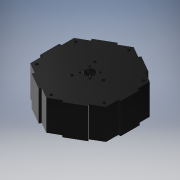
# Autodesk Inventor part: Spur Gear2
Saved by Autodesk Inventor 2017 (Build 210142000, 142)
## iProperties
Created: 2018-10-09
Part Number: Spur Gear2
Material: ABS Plastic
Document SubType Name: Modeling
Designer: Zach
Categories: <?xml version="1.0" encoding="UTF-16"?> <MemberInstance><Categories><FamilyTemplate><FamilyTemplateParameter ValueType="xs:double" Id="1" ObjectReferenceKey="da_z" ObjectType="kUserParameterObject"/><FamilyTemplateParameter ValueType="xs:double" Id="2" ObjectReferenceKey="da_b" ObjectType="kUserParameterObject"/><FamilyTemplateParameter ValueType="xs:double" Id="3" ObjectReferenceKey="da_beta" ObjectType="kUserParameterObject"/><FamilyTemplateParameter ValueType="xs:double" Id="4" ObjectReferenceKey="da_da" ObjectType="kUserParameterObject"/><FamilyTemplateParameter ValueType="xs:double" Id="5" ObjectReferenceKey="da_aw" ObjectType="kUserParameterObject"/><FamilyTemplateParameter ValueType="xs:string" Id="6" ObjectReferenceKey="EAIAABAAAACIAQAAAAAAAIAAAAAAAAAA" ObjectType="83910656" SubObjectId="SurfaceGeometry"/></FamilyTemplate><ParamToTemplateMap><ParamToTemplate CategoryParameter="//CategoryParameter[@InternalName='046C89C9-8512-4d59-83FE-43B91F4F132A']" TemplateParameter="1"/><ParamToTemplate CategoryParameter="//CategoryParameter[@InternalName='2552DF32-E462-4b46-AEBF-C6C7768E72AC']" TemplateParameter="2"/><ParamToTemplate CategoryParameter="//CategoryParameter[@InternalName='C9EE641D-15FC-4fae-A226-E94C4372FDD7']" TemplateParameter="3"/><ParamToTemplate><ParamToTemplate CategoryParameter="//CategoryParameter[@InternalName='00B6519A-459B-49c7-AD84-2E56D39A5744']" ConstantValue="0.000000"/></ParamToTemplate><ParamToTemplate><ParamToTemplate CategoryParameter="//CategoryParameter[@InternalName='04B31F0E-C7A6-4894-AA32-9629BEFACF47']" ConstantValue="1.000000"/></ParamToTemplate><ParamToTemplate><ParamToTemplate CategoryParameter="//CategoryParameter[@InternalName='43CBEC2E-7847-49e7-A936-2F7889FCB2D9']" ConstantValue="0.250000"/></ParamToTemplate><ParamToTemplate><ParamToTemplate CategoryParameter="//CategoryParameter[@InternalName='B1EFC894-105D-4ebd-86BF-FA20ED196853']" ConstantValue="0.350000"/></ParamToTemplate><ParamToTemplate><ParamToTemplate CategoryParameter="//CategoryParameter[@InternalName='51175063-3D10-4879-93E8-6246FE8B403D']" ConstantValue="2060000000.000000"/></ParamToTemplate><ParamToTemplate><ParamToTemplate CategoryParameter="//CategoryParameter[@InternalName='A3A52E27-4454-46a9-B0BD-C932399B70AF']" ConstantValue="0.300000"/></ParamToTemplate><ParamToTemplate><ParamToTemplate CategoryParameter="//CategoryParameter[@InternalName='91B76062-C214-41d9-B1B9-14D2AB99603D']" ConstantValue="0.200000"/></ParamToTemplate><ParamToTemplate><ParamToTemplate CategoryParameter="//CategoryParameter[@InternalName='374E806E-8B8A-4dda-A9AA-1039D6500AD2']" ConstantValue="5.000000"/></ParamToTemplate><ParamToTemplate><ParamToTemplate CategoryParameter="//CategoryParameter[@InternalName='2D373A89-B862-43d6-8D0B-0CBF12AB9F6C']" ConstantValue="0.392699"/></ParamToTemplate><ParamToTemplate CategoryParameter="//CategoryParameter[@InternalName='37777632-D6A2-4fac-9D53-DB8ACD95C989']" TemplateParameter="4"/><ParamToTemplate CategoryParameter="//CategoryParameter[@InternalName='FD1017F1-B727-4f7e-9707-0F86F1FF9423']" TemplateParameter="5"/><ParamToTemplate><ParamToTemplate CategoryParameter="//CategoryParameter[@InternalName='9E1B4470-B2D3-4ff1-B813-535BB4CDF51A']" ConstantValue="3520000.000000"/></ParamToTemplate><ParamToTemplate><ParamToTemplate CategoryParameter="//CategoryParameter[@InternalName='F8452263-BFF6-458c-9FB1-07C4B99E95CD']" ConstantValue="11400000.000000"/></ParamToTemplate><ParamToTemplate><ParamToTemplate CategoryParameter="//CategoryParameter[@InternalName='3E3BB259-FD49-497f-8171-6EBC954A3479']" ConstantValue="2.000000"/></ParamToTemplate><ParamToTemplate CategoryParameter="//CategoryParameter[@InternalName='27C3BAF2-7550-4e4b-AE2C-0DB134B7D9B7']" TemplateParameter="6"/></ParamToTemplateMap><Category DisplayName="Gear" InternalName="DC85795E-93AB-48d5-8EEE-5A27447B64BD" Mnemonic="Gear"><CategoryParameter DisplayName="z" InternalName="046C89C9-8512-4d59-83FE-43B91F4F132A" Mnemonic="z"/><CategoryParameter DisplayName="b" InternalName="2552DF32-E462-4b46-AEBF-C6C7768E72AC" Mnemonic="b"/><CategoryParameter DisplayName="||b|" InternalName="C9EE641D-15FC-4fae-A226-E94C4372FDD7" Mnemonic="beta"/><CategoryParameter DisplayName="x" InternalName="00B6519A-459B-49c7-AD84-2E56D39A5744" Mnemonic="x"/><CategoryParameter DisplayName="a*" InternalName="04B31F0E-C7A6-4894-AA32-9629BEFACF47" Mnemonic="a"/><CategoryParameter DisplayName="c*" InternalName="43CBEC2E-7847-49e7-A936-2F7889FCB2D9" Mnemonic="c"/><CategoryParameter DisplayName="r|.f|*" InternalName="B1EFC894-105D-4ebd-86BF-FA20ED196853" Mnemonic="rf"/><CategoryParameter DisplayName="E" InternalName="51175063-3D10-4879-93E8-6246FE8B403D" Mnemonic="E"/><CategoryParameter DisplayName="||m|" InternalName="A3A52E27-4454-46a9-B0BD-C932399B70AF" Mnemonic="mi"/><Category DisplayName="SpurGear" InternalName="26C5A22E-A91E-4dfd-A3B3-23CCAFAE1764" Mnemonic="SpurGear"><CategoryParameter DisplayName="m" InternalName="91B76062-C214-41d9-B1B9-14D2AB99603D" Mnemonic="m"/><CategoryParameter DisplayName="P" InternalName="374E806E-8B8A-4dda-A9AA-1039D6500AD2" Mnemonic="PP"/><CategoryParameter DisplayName="||a|" InternalName="2D373A89-B862-43d6-8D0B-0CBF12AB9F6C" Mnemonic="alpha"/><CategoryParameter DisplayName="d|.a|" InternalName="37777632-D6A2-4fac-9D53-DB8ACD95C989" Mnemonic="da"/><CategoryParameter DisplayName="a|.w|" InternalName="FD1017F1-B727-4f7e-9707-0F86F1FF9423" Mnemonic="aw"/><CategoryParameter DisplayName="||s||.Flim|" InternalName="9E1B4470-B2D3-4ff1-B813-535BB4CDF51A" Mnemonic="sFlim"/><CategoryParameter DisplayName="||s||.Hlim|" InternalName="F8452263-BFF6-458c-9FB1-07C4B99E95CD" Mnemonic="sHlim"/><CategoryParameter DisplayName="type" InternalName="3E3BB259-FD49-497f-8171-6EBC954A3479" Mnemonic="type"/><Category DisplayName="InternalSpurGear" InternalName="7CF704F6-14A9-42f8-93CE-E71DF57C2B55" Mnemonic="InternalSpurGear"><CategoryParameter DisplayName="PitchDiameter" InternalName="27C3BAF2-7550-4e4b-AE2C-0DB134B7D9B7" Mnemonic="IDS_PITCHDIAM"/></Category></Category></Category></Categories></MemberInstance>
Density: 1.06 g/cm^3
Appearance: Smooth - Black
Mass: 196.31 g
Surface Area: 506.785 cm^2
Volume: 185.198 cm^3
CustomPartVersion: 0
Author: Zach
Autodesk Inventor part; units mm, degrees
ref_plane "YZ Plane" through (0, 0, 0) normal (1, 0, 0) x (0, 1, 0)
ref_plane "XZ Plane" through (0, 0, 0) normal (0, 1, 0) x (-1, 0, 0)
ref_plane "XY Plane" through (0, 0, 0) normal (0, 0, 1) x (1, 0, 0)
sketch "Sketch1" plane through (0, 0, 0) normal (0, 0, 1) x (1, 0, 0)
  circle A0 centre (0, 0) radius 52.25
  dimension "d0" = 104.5
  constraints: 1 centre point
  measures "d0" diameter of A0
extrude "Extrusion1" add sketch "Sketch1" along normal blind 10
ref_plane "Work Plane2" through (0, 0, 5) normal (0, 0, 1) x (1, 0, 0)
sketch "Sketch2" plane through (0, 0, 0) normal (0, 0, -1) x (-1, 0, 0)
  circle A0 centre (0, 0) radius 52.25 projected
  circle A1 centre (0, 0) radius 45
  dimension "d3" = 90
  constraints: 1 centre point, 1 coincident
  measures "d3" diameter of A1
surface extrude "Pitch Diameter" sketch "Sketch2" against normal through all shown no curves A1
ref_plane "Work Plane8" through (0, 0, 0) normal (0.9975641, 0.0697565, 0) x (0, 0, 1)
ref_plane "Work Plane9" through (0, 0, 0) normal (1, 0, 0) x (0, 1, 0)
spur gear teeth "Spur Gear" teeth 45 pitch diameter 90 tip diameter 86.2612 root diameter 95 face width 10 start plane through (0, 0, 0) normal (0, 0, -1) x (-1, 0, 0)
sketch "Sketch3" plane through (0, 0, 10) normal (0, 0, 1) x (1, 0, 0)
  arc A0 (2.2573, -43.0715) -> (3.7591, -42.9665) centre (0, 0) ccw projected
  arc A1 (0.829, -47.4928) -> (2.2573, -43.0715) centre (-19.4558, -38.4984) ccw projected
  arc A2 (-0.829, -47.4928) -> (0.829, -47.4928) centre (0, 0) ccw projected
  arc A3 (-2.2573, -43.0715) -> (-0.829, -47.4928) centre (19.4558, -38.4984) ccw projected
  arc A4 (-3.7591, -42.9665) -> (-2.2573, -43.0715) centre (0, 0) ccw projected
  arc A5 (-5.7888, -47.1459) -> (-3.7591, -42.9665) centre (-24.6244, -35.4161) ccw projected
  arc A6 (-7.4306, -46.9152) -> (-5.7888, -47.1459) centre (0, 0) ccw projected
  arc A7 (-8.2297, -42.3382) -> (-7.4306, -46.9152) centre (13.9085, -40.8315) ccw projected
  arc A8 (-9.7023, -42.0252) -> (-8.2297, -42.3382) centre (0, 0) ccw projected
  arc A9 (-12.2939, -45.8815) -> (-9.7023, -42.0252) centre (-29.3137, -31.6443) ccw projected
  arc A10 (-13.8877, -45.4245) -> (-12.2939, -45.8815) centre (0, 0) ccw projected
  arc A11 (-14.0419, -40.7808) -> (-13.8877, -45.4245) centre (8.0905, -42.3698) ccw projected
  arc A12 (-15.4566, -40.2659) -> (-14.0419, -40.7808) centre (0, 0) ccw projected
  arc A13 (-18.5597, -43.724) -> (-15.4566, -40.2659) centre (-33.4325, -27.2567) ccw projected
  arc A14 (-20.0744, -43.0496) -> (-18.5597, -43.724) centre (0, 0) ccw projected
  arc A15 (-19.5809, -38.4296) -> (-20.0744, -43.0496) centre (2.115, -43.0835) ccw projected
  arc A16 (-20.9101, -37.7229) -> (-19.5809, -38.4296) centre (0, 0) ccw projected
  arc A17 (-24.4643, -40.7154) -> (-20.9101, -37.7229) centre (-36.9005, -22.3385) ccw projected
  arc A18 (-25.8704, -39.8369) -> (-24.4643, -40.7154) centre (0, 0) ccw projected
  arc A19 (-24.7387, -35.3305) -> (-25.8704, -39.8369) centre (-3.9016, -42.9585) ccw projected
  arc A20 (-25.9566, -34.4456) -> (-24.7387, -35.3305) centre (0, 0) ccw projected
  arc A21 (-29.8927, -36.9144) -> (-25.9566, -34.4456) centre (-39.6503, -16.9856) ccw projected
  arc A22 (-31.1628, -35.8487) -> (-29.8927, -36.9144) centre (0, 0) ccw projected
  arc A23 (-29.415, -31.5437) -> (-31.1628, -35.8487) centre (-9.8423, -41.9975) ccw projected
  arc A24 (-30.4979, -30.4979) -> (-29.415, -31.5437) centre (0, 0) ccw projected
  arc A25 (-34.7393, -32.3949) -> (-30.4979, -30.4979) centre (-41.6284, -11.302) ccw projected
  arc A26 (-35.8487, -31.1628) -> (-34.7393, -32.3949) centre (0, 0) ccw projected
  arc A27 (-33.5188, -27.143) -> (-35.8487, -31.1628) centre (-15.5915, -40.219) ccw projected
  arc A28 (-34.4456, -25.9566) -> (-33.5188, -27.143) centre (0, 0) ccw projected
  arc A29 (-38.9097, -27.2449) -> (-34.4456, -25.9566) centre (-42.7962, -5.3985) ccw projected
  arc A30 (-39.8369, -25.8704) -> (-38.9097, -27.2449) centre (0, 0) ccw projected
  arc A31 (-36.9701, -22.2139) -> (-39.8369, -25.8704) centre (-21.0371, -37.6576) ccw projected
  arc A32 (-37.7229, -20.9101) -> (-36.9701, -22.2139) centre (0, 0) ccw projected
  arc A33 (-42.3228, -21.5645) -> (-37.7229, -20.9101) centre (-43.131, 0.6101) ccw projected
  arc A34 (-43.0496, -20.0744) -> (-42.3228, -21.5645) centre (0, 0) ccw projected
  arc A35 (-39.7019, -16.8525) -> (-43.0496, -20.0744) centre (-26.0733, -34.3634) ccw projected
  arc A36 (-40.2659, -15.4566) -> (-39.7019, -16.8525) centre (0, 0) ccw projected
  arc A37 (-44.9121, -15.4645) -> (-40.2659, -15.4566) centre (-42.6264, 6.6069) ccw projected
  arc A38 (-45.4245, -13.8877) -> (-44.9121, -15.4645) centre (0, 0) ccw projected
  arc A39 (-41.6609, -11.163) -> (-45.4245, -13.8877) centre (-30.602, -30.4002) ccw projected
  arc A40 (-42.0252, -9.7023) -> (-41.6609, -11.163) centre (0, 0) ccw projected
  arc A41 (-46.6273, -9.0634) -> (-42.0252, -9.7023) centre (-41.292, 12.475) ccw projected
  arc A42 (-46.9152, -7.4306) -> (-46.6273, -9.0634) centre (0, 0) ccw projected
  arc A43 (-42.8091, -5.2563) -> (-46.9152, -7.4306) centre (-34.5351, -25.8454) ccw projected
  arc A44 (-42.9665, -3.7591) -> (-42.8091, -5.2563) centre (0, 0) ccw projected
  arc A45 (-47.4349, -2.486) -> (-42.9665, -3.7591) centre (-39.154, 18.1004) ccw projected
  arc A46 (-47.4928, -0.829) -> (-47.4349, -2.486) centre (0, 0) ccw projected
  arc A47 (-43.124, 0.7527) -> (-47.4928, -0.829) centre (-37.796, -20.7875) ccw projected
  arc A48 (-43.0715, 2.2573) -> (-43.124, 0.7527) centre (0, 0) ccw projected
  arc A49 (-47.3192, 4.1399) -> (-43.0715, 2.2573) centre (-36.2539, 23.3734) ccw projected
  arc A50 (-47.1459, 5.7888) -> (-47.3192, 4.1399) centre (0, 0) ccw projected
  arc A51 (-42.5996, 6.7471) -> (-47.1459, 5.7888) centre (-40.3212, -15.325) ccw projected
  arc A52 (-42.3382, 8.2297) -> (-42.5996, 6.7471) centre (0, 0) ccw projected
  arc A53 (-46.2826, 10.6852) -> (-42.3382, 8.2297) centre (-32.6481, 28.1915) ccw projected
  arc A54 (-45.8815, 12.2939) -> (-46.2826, 10.6852) centre (0, 0) ccw projected
  arc A55 (-41.246, 12.6102) -> (-45.8815, 12.2939) centre (-42.0617, -9.5642) ccw projected
  arc A56 (-40.7808, 14.0419) -> (-41.246, 12.6102) centre (0, 0) ccw projected
  arc A57 (-44.3451, 17.0225) -> (-40.7808, 14.0419) centre (-28.4069, 32.4609) ccw projected
  arc A58 (-43.724, 18.5597) -> (-44.3451, 17.0225) centre (0, 0) ccw projected
  arc A59 (-39.0896, 18.2278) -> (-43.724, 18.5597) centre (-42.9834, -3.6173) ccw projected
  arc A60 (-38.4296, 19.5809) -> (-39.0896, 18.2278) centre (0, 0) ccw projected
  arc A61 (-41.5444, 23.0285) -> (-38.4296, 19.5809) centre (-23.6127, 36.0984) ccw projected
  arc A62 (-40.7154, 24.4643) -> (-41.5444, 23.0285) centre (0, 0) ccw projected
  arc A63 (-36.1724, 23.4906) -> (-40.7154, 24.4643) centre (-43.0685, 2.4) ccw projected
  arc A64 (-35.3305, 24.7387) -> (-36.1724, 23.4906) centre (0, 0) ccw projected
  arc A65 (-37.9352, 28.5862) -> (-35.3305, 24.7387) centre (-18.359, 39.0334) ccw projected
  arc A66 (-36.9144, 29.8927) -> (-37.9352, 28.5862) centre (0, 0) ccw projected
  arc A67 (-32.5511, 28.2962) -> (-36.9144, 29.8927) centre (-42.3154, 8.3706) ccw projected
  arc A68 (-31.5437, 29.415) -> (-32.5511, 28.2962) centre (0, 0) ccw projected
  arc A69 (-33.5876, 33.5876) -> (-31.5437, 29.415) centre (-12.748, 41.2086) ccw projected
  arc A70 (-32.3949, 34.7393) -> (-33.5876, 33.5876) centre (0, 0) ccw projected
  arc A71 (-28.2962, 32.5511) -> (-32.3949, 34.7393) centre (-40.7386, 14.1783) ccw projected
  arc A72 (-27.143, 33.5188) -> (-28.2962, 32.5511) centre (0, 0) ccw projected
  arc A73 (-28.5862, 37.9352) -> (-27.143, 33.5188) centre (-6.8888, 42.5817) ccw projected
  arc A74 (-27.2449, 38.9097) -> (-28.5862, 37.9352) centre (0, 0) ccw projected
  arc A75 (-23.4906, 36.1724) -> (-27.2449, 38.9097) centre (-38.3689, 19.7101) ccw projected
  arc A76 (-22.2139, 36.9701) -> (-23.4906, 36.1724) centre (0, 0) ccw projected
  arc A77 (-23.0285, 41.5444) -> (-22.2139, 36.9701) centre (-0.8955, 43.126) ccw projected
  arc A78 (-21.5645, 42.3228) -> (-23.0285, 41.5444) centre (0, 0) ccw projected
  arc A79 (-18.2278, 39.0896) -> (-21.5645, 42.3228) centre (-35.2524, 24.8582) ccw projected
  arc A80 (-16.8525, 39.7019) -> (-18.2278, 39.0896) centre (0, 0) ccw projected
  arc A81 (-17.0225, 44.3451) -> (-16.8525, 39.7019) centre (5.1152, 42.831) ccw projected
  arc A82 (-15.4645, 44.9121) -> (-17.0225, 44.3451) centre (0, 0) ccw projected
  arc A83 (-12.6102, 41.246) -> (-15.4645, 44.9121) centre (-31.4497, 29.5224) ccw projected
  arc A84 (-11.163, 41.6609) -> (-12.6102, 41.246) centre (0, 0) ccw projected
  arc A85 (-10.6852, 46.2826) -> (-11.163, 41.6609) centre (11.0263, 41.7022) ccw projected
  arc A86 (-9.0634, 46.6273) -> (-10.6852, 46.2826) centre (0, 0) ccw projected
  arc A87 (-6.7471, 42.5996) -> (-9.0634, 46.6273) centre (-27.0349, 33.6121) ccw projected
  arc A88 (-5.2563, 42.8091) -> (-6.7471, 42.5996) centre (0, 0) ccw projected
  arc A89 (-4.1399, 47.3192) -> (-5.2563, 42.8091) centre (16.7229, 39.7618) ccw projected
  arc A90 (-2.486, 47.4349) -> (-4.1399, 47.3192) centre (0, 0) ccw projected
  arc A91 (-0.7527, 43.124) -> (-2.486, 47.4349) centre (-22.0939, 37.0475) ccw projected
  arc A92 (0.7527, 43.124) -> (-0.7527, 43.124) centre (0, 0) ccw projected
  arc A93 (2.486, 47.4349) -> (0.7527, 43.124) centre (22.0939, 37.0475) ccw projected
  arc A94 (4.1399, 47.3192) -> (2.486, 47.4349) centre (0, 0) ccw projected
  arc A95 (5.2563, 42.8091) -> (4.1399, 47.3192) centre (-16.7229, 39.7618) ccw projected
  arc A96 (6.7471, 42.5996) -> (5.2563, 42.8091) centre (0, 0) ccw projected
  arc A97 (9.0634, 46.6273) -> (6.7471, 42.5996) centre (27.0349, 33.6121) ccw projected
  arc A98 (10.6852, 46.2826) -> (9.0634, 46.6273) centre (0, 0) ccw projected
  arc A99 (11.163, 41.6609) -> (10.6852, 46.2826) centre (-11.0263, 41.7022) ccw projected
  arc A100 (12.6102, 41.246) -> (11.163, 41.6609) centre (0, 0) ccw projected
  arc A101 (15.4645, 44.9121) -> (12.6102, 41.246) centre (31.4497, 29.5224) ccw projected
  arc A102 (17.0225, 44.3451) -> (15.4645, 44.9121) centre (0, 0) ccw projected
  arc A103 (16.8525, 39.7019) -> (17.0225, 44.3451) centre (-5.1152, 42.831) ccw projected
  arc A104 (18.2278, 39.0896) -> (16.8525, 39.7019) centre (0, 0) ccw projected
  arc A105 (21.5645, 42.3228) -> (18.2278, 39.0896) centre (35.2524, 24.8582) ccw projected
  arc A106 (23.0285, 41.5444) -> (21.5645, 42.3228) centre (0, 0) ccw projected
  arc A107 (22.2139, 36.9701) -> (23.0285, 41.5444) centre (0.8955, 43.126) ccw projected
  arc A108 (23.4906, 36.1724) -> (22.2139, 36.9701) centre (0, 0) ccw projected
  arc A109 (27.2449, 38.9097) -> (23.4906, 36.1724) centre (38.3689, 19.7101) ccw projected
  arc A110 (28.5862, 37.9352) -> (27.2449, 38.9097) centre (0, 0) ccw projected
  arc A111 (27.143, 33.5188) -> (28.5862, 37.9352) centre (6.8888, 42.5817) ccw projected
  arc A112 (28.2962, 32.5511) -> (27.143, 33.5188) centre (0, 0) ccw projected
  arc A113 (32.3949, 34.7393) -> (28.2962, 32.5511) centre (40.7386, 14.1783) ccw projected
  arc A114 (33.5876, 33.5876) -> (32.3949, 34.7393) centre (0, 0) ccw projected
  arc A115 (31.5437, 29.415) -> (33.5876, 33.5876) centre (12.748, 41.2086) ccw projected
  arc A116 (32.5511, 28.2962) -> (31.5437, 29.415) centre (0, 0) ccw projected
  arc A117 (36.9144, 29.8927) -> (32.5511, 28.2962) centre (42.3154, 8.3706) ccw projected
  arc A118 (37.9352, 28.5862) -> (36.9144, 29.8927) centre (0, 0) ccw projected
  arc A119 (35.3305, 24.7387) -> (37.9352, 28.5862) centre (18.359, 39.0334) ccw projected
  arc A120 (36.1724, 23.4906) -> (35.3305, 24.7387) centre (0, 0) ccw projected
  arc A121 (40.7154, 24.4643) -> (36.1724, 23.4906) centre (43.0685, 2.4) ccw projected
  arc A122 (41.5444, 23.0285) -> (40.7154, 24.4643) centre (0, 0) ccw projected
  arc A123 (38.4296, 19.5809) -> (41.5444, 23.0285) centre (23.6127, 36.0984) ccw projected
  arc A124 (39.0896, 18.2278) -> (38.4296, 19.5809) centre (0, 0) ccw projected
  arc A125 (43.724, 18.5597) -> (39.0896, 18.2278) centre (42.9834, -3.6173) ccw projected
  arc A126 (44.3451, 17.0225) -> (43.724, 18.5597) centre (0, 0) ccw projected
  arc A127 (40.7808, 14.0419) -> (44.3451, 17.0225) centre (28.4069, 32.4609) ccw projected
  arc A128 (41.246, 12.6102) -> (40.7808, 14.0419) centre (0, 0) ccw projected
  arc A129 (45.8815, 12.2939) -> (41.246, 12.6102) centre (42.0617, -9.5642) ccw projected
  arc A130 (46.2826, 10.6852) -> (45.8815, 12.2939) centre (0, 0) ccw projected
  arc A131 (42.3382, 8.2297) -> (46.2826, 10.6852) centre (32.6481, 28.1915) ccw projected
  arc A132 (42.5996, 6.7471) -> (42.3382, 8.2297) centre (0, 0) ccw projected
  arc A133 (47.1459, 5.7888) -> (42.5996, 6.7471) centre (40.3212, -15.325) ccw projected
  arc A134 (47.3192, 4.1399) -> (47.1459, 5.7888) centre (0, 0) ccw projected
  arc A135 (43.0715, 2.2573) -> (47.3192, 4.1399) centre (36.2539, 23.3734) ccw projected
  arc A136 (43.124, 0.7527) -> (43.0715, 2.2573) centre (0, 0) ccw projected
  arc A137 (47.4928, -0.829) -> (43.124, 0.7527) centre (37.796, -20.7875) ccw projected
  arc A138 (47.4349, -2.486) -> (47.4928, -0.829) centre (0, 0) ccw projected
  arc A139 (42.9665, -3.7591) -> (47.4349, -2.486) centre (39.154, 18.1004) ccw projected
  arc A140 (42.8091, -5.2563) -> (42.9665, -3.7591) centre (0, 0) ccw projected
  arc A141 (46.9152, -7.4306) -> (42.8091, -5.2563) centre (34.5351, -25.8454) ccw projected
  arc A142 (46.6273, -9.0634) -> (46.9152, -7.4306) centre (0, 0) ccw projected
  arc A143 (42.0252, -9.7023) -> (46.6273, -9.0634) centre (41.292, 12.475) ccw projected
  arc A144 (41.6609, -11.163) -> (42.0252, -9.7023) centre (0, 0) ccw projected
  arc A145 (45.4245, -13.8877) -> (41.6609, -11.163) centre (30.602, -30.4002) ccw projected
  arc A146 (44.9121, -15.4645) -> (45.4245, -13.8877) centre (0, 0) ccw projected
  arc A147 (40.2659, -15.4566) -> (44.9121, -15.4645) centre (42.6264, 6.6069) ccw projected
  arc A148 (39.7019, -16.8525) -> (40.2659, -15.4566) centre (0, 0) ccw projected
  arc A149 (43.0496, -20.0744) -> (39.7019, -16.8525) centre (26.0733, -34.3634) ccw projected
  arc A150 (42.3228, -21.5645) -> (43.0496, -20.0744) centre (0, 0) ccw projected
  arc A151 (37.7229, -20.9101) -> (42.3228, -21.5645) centre (43.131, 0.6101) ccw projected
  arc A152 (36.9701, -22.2139) -> (37.7229, -20.9101) centre (0, 0) ccw projected
  arc A153 (39.8369, -25.8704) -> (36.9701, -22.2139) centre (21.0371, -37.6576) ccw projected
  arc A154 (38.9097, -27.2449) -> (39.8369, -25.8704) centre (0, 0) ccw projected
  arc A155 (34.4456, -25.9566) -> (38.9097, -27.2449) centre (42.7962, -5.3985) ccw projected
  arc A156 (33.5188, -27.143) -> (34.4456, -25.9566) centre (0, 0) ccw projected
  arc A157 (35.8487, -31.1628) -> (33.5188, -27.143) centre (15.5915, -40.219) ccw projected
  arc A158 (34.7393, -32.3949) -> (35.8487, -31.1628) centre (0, 0) ccw projected
  arc A159 (30.4979, -30.4979) -> (34.7393, -32.3949) centre (41.6284, -11.302) ccw projected
  arc A160 (29.415, -31.5437) -> (30.4979, -30.4979) centre (0, 0) ccw projected
  arc A161 (31.1628, -35.8487) -> (29.415, -31.5437) centre (9.8423, -41.9975) ccw projected
  arc A162 (29.8927, -36.9144) -> (31.1628, -35.8487) centre (0, 0) ccw projected
  arc A163 (25.9566, -34.4456) -> (29.8927, -36.9144) centre (39.6503, -16.9856) ccw projected
  arc A164 (24.7387, -35.3305) -> (25.9566, -34.4456) centre (0, 0) ccw projected
  arc A165 (25.8704, -39.8369) -> (24.7387, -35.3305) centre (3.9016, -42.9585) ccw projected
  arc A166 (24.4643, -40.7154) -> (25.8704, -39.8369) centre (0, 0) ccw projected
  arc A167 (20.9101, -37.7229) -> (24.4643, -40.7154) centre (36.9005, -22.3385) ccw projected
  arc A168 (19.5809, -38.4296) -> (20.9101, -37.7229) centre (0, 0) ccw projected
  arc A169 (20.0744, -43.0496) -> (19.5809, -38.4296) centre (-2.115, -43.0835) ccw projected
  arc A170 (18.5597, -43.724) -> (20.0744, -43.0496) centre (0, 0) ccw projected
  arc A171 (15.4566, -40.2659) -> (18.5597, -43.724) centre (33.4325, -27.2567) ccw projected
  arc A172 (14.0419, -40.7808) -> (15.4566, -40.2659) centre (0, 0) ccw projected
  arc A173 (13.8877, -45.4245) -> (14.0419, -40.7808) centre (-8.0905, -42.3698) ccw projected
  arc A174 (12.2939, -45.8815) -> (13.8877, -45.4245) centre (0, 0) ccw projected
  arc A175 (9.7023, -42.0252) -> (12.2939, -45.8815) centre (29.3137, -31.6443) ccw projected
  arc A176 (8.2297, -42.3382) -> (9.7023, -42.0252) centre (0, 0) ccw projected
  arc A177 (7.4306, -46.9152) -> (8.2297, -42.3382) centre (-13.9085, -40.8315) ccw projected
  arc A178 (5.7888, -47.1459) -> (7.4306, -46.9152) centre (0, 0) ccw projected
  arc A179 (3.7591, -42.9665) -> (5.7888, -47.1459) centre (24.6244, -35.4161) ccw projected
  circle A180 centre (0, 0) radius 52.25 projected
extrude "Extrusion2" add sketch "Sketch3" along normal blind 15
sketch "Sketch4" plane through (0, 0, 25) normal (0, 0, 1) x (1, 0, 0)
  circle A0 centre (0, 0) radius 52.25 projected
  circle A1 centre (0, 0) radius 6.75
  circle A2 centre (30, 0) radius 3
  circle A3 centre (15, 25.9808) radius 3
  circle A4 centre (-15, 25.9808) radius 3
  circle A5 centre (-30, 0) radius 3
  circle A6 centre (-15, -25.9808) radius 3
  circle A7 centre (15, -25.9808) radius 3
  dimension "d55" = 13.5
  dimension "d56" = 6
  dimension "d57" = 30
  dimension "d60" = 360
  constraints: 7 centre point, 1 coincident, 1 horizontal alignment, 13 other
  measures "d55" diameter of A1
  measures "d56" diameter of A2
  measures "d57" distance of A2.centre point (0, 0)
extrude "Extrusion3" add sketch "Sketch4" along normal blind 15 contours A0 | A2 | A3 | A4 | A5 | A6 | A7
sketch "Sketch11" plane through (0, 0, 40) normal (0, 0, 1) x (1, 0, 0)
  circle A0 centre (0, 0) radius 52.25 projected
  circle A1 centre (0, 0) radius 57.5
  dimension "d96" = 115
  constraints: 1 centre point, 1 coincident
  measures "d96" diameter of A1
extrude "Extrusion9" add sketch "Sketch11" against normal blind 39.9
sketch "Sketch12" plane through (0, 0, 40) normal (0, 0, 1) x (1, 0, 0)
  circle A0 centre (0, 0) radius 6.75 projected
  line L0 (0, 57.5) -> (49.7965, 28.75)
  line L1 (49.7965, 28.75) -> (49.7965, -28.75)
  line L2 (49.7965, -28.75) -> (0, -57.5)
  line L3 (0, -57.5) -> (-49.7965, -28.75)
  line L4 (-49.7965, -28.75) -> (-49.7965, 28.75)
  line L5 (-49.7965, 28.75) -> (0, 57.5)
  circle A1 centre (0, 0) radius 57.5 projected
  constraints: 12 end point, 2 coincident, 2 vertical alignment, 14 other
extrude "Extrusion10" cut sketch "Sketch12" against normal through all contours A1 L0 | L5 A1 | A1 L1 | L4 A1 | A1 L2 | L3 A1
sketch "Sketch18" plane through (0, 0, 40) normal (0, 0, 1) x (1, 0, 0)
  circle A0 centre (17.5, 0) radius 2
  circle A1 centre (-8.75, 15.1554) radius 2
  circle A2 centre (-8.75, -15.1554) radius 2
  point P0 (0, 0)
  dimension "d133" = 4
  dimension "d134" = 17.5
  dimension "d137" = 360
  constraints: 3 centre point, 1 horizontal alignment, 7 other
  measures "d133" diameter of A0
  measures "d134" distance of point (0, 0) A0.centre
extrude "Extrusion15" cut sketch "Sketch18" against normal through all
sketch "Sketch20" plane through (0, 0, 40) normal (0, 0, 1) x (1, 0, 0)
  circle A0 centre (0, 51) radius 2
  circle A1 centre (-44.1673, 25.5) radius 2
  circle A2 centre (-44.1673, -25.5) radius 2
  circle A3 centre (0, -51) radius 2
  circle A4 centre (44.1673, -25.5) radius 2
  circle A5 centre (44.1673, 25.5) radius 2
  circle A6 centre (0, 0) radius 6.75 projected
  line L0 (0, -51) -> (0, 51)
  dimension "d155" = 4
  dimension "d159" = 360
  dimension "d198" = 102
  constraints: 6 centre point, 2 end point, 1 coincident, 1 vertical, 13 other
  measures "d155" diameter of A0
  measures "d198" distance of L0.start L0.end
extrude "Extrusion17" cut sketch "Sketch20" against normal through all contours A0 | A1 | A2 | A3 | A4 | A5
sketch "Sketch28" plane through (0, 0, 25) normal (0, 0, -1) x (-1, 0, 0)
  circle A0 centre (0, 0) radius 6.75 projected
  circle A1 centre (0, 0) radius 11
  dimension "d186" = 22
  constraints: 1 centre point, 1 coincident
  measures "d186" diameter of A1
extrude "Extrusion24" add sketch "Sketch28" along normal blind 20
sketch "Sketch29" plane through (0, 0, 40) normal (0, 0, 1) x (1, 0, 0)
  circle A0 centre (0, 0) radius 13
  dimension "d189" = 26
  constraints: 1 centre point, 1 coincident
  measures "d189" diameter of A0
extrude "Extrusion25" cut sketch "Sketch29" against normal blind 11.1
sketch "Sketch30" plane through (0, 0, 0) normal (1, 0, 0) x (0, 1, 0)
  circle A0 centre (0, 34.45) radius 4
  line L0 (-13, 40) -> (13, 40) projected
  point P0 (0, 0)
  point P1 (0, 40)
  dimension "d192" = 8
  dimension "d195" = 5.55
  constraints: 1 centre point, 1 midpoint, 1 vertical alignment
  measures "d192" diameter of A0
  measures "d195" distance from line of L0 A0.centre
extrude "Extrusion26" cut sketch "Sketch30" against normal through all
sketch "Sketch31" plane through (0, 0, 40) normal (0, 0, 1) x (1, 0, 0)
  line L0 (-49.7965, -4) -> (-49.7965, 4) projected
  line L1 (-49.7965, -4) -> (-3.0859, -4)
  line L2 (-3.0859, -4) -> (-3.0859, 4)
  line L3 (-3.0859, 4) -> (-49.7965, 4)
  line L4 (-49.7965, 4) -> (-49.7965, -4)
  point P0 (0, 0)
  constraints: 8 end point, 2 parallel, 1 horizontal, 1 perpendicular
extrude "Extrusion27" cut sketch "Sketch31" against normal blind 5.55
sketch "Sketch32" plane through (-49.7965, 28.75, 40) normal (-0.5, 0.8660254, 0) x (0.8660254, 0.5, 0)
  line L0 (41.25, 40) -> (16.25, 40)
  line L1 (16.25, 40) -> (16.25, 0)
  line L2 (16.25, 0) -> (41.25, 0)
  line L3 (41.25, 0) -> (41.25, 40)
  line L4 (57.5, 0) -> (0, 0) projected
  line L5 (12.9268, 40) -> (44.5732, 40) projected
  point P0 (28.75, 40)
  point P1 (28.75, 0)
  point P2 (28.75, 40)
  dimension "d199" = 25
  constraints: 8 end point, 4 midpoint, 2 parallel, 1 horizontal, 1 perpendicular
  measures "d199" distance between parallel lines of L1 L3
extrude "Extrusion28" add sketch "Sketch32" along normal blind 3
pattern_circular "Circular Pattern4" count 6 over 360 about axis through (0, 0, 0) along (0, 0, 1) of "Extrusion28"
sketch "Sketch33" plane through (-49.7965, -4, 40) normal (1, 0, 0) x (0, 0, -1)
  line L0 (5.55, 8) -> (0, 8) projected
  line L1 (0, 0) -> (0, 8) projected
  line L2 (0, 0) -> (5.55, 0) projected
  arc A0 (5.55, 0) -> (5.55, 8) centre (5.55, 4) ccw projected
  point P0 (40, 4)
extrude "Extrusion29" cut sketch "Sketch33" against normal through all
ref_plane "Work Plane11" through (0, 0, 10) normal (0, 0, -1) x (-1, 0, 0)
sketch "Sketch34" plane through (0, 0, 10) normal (0, 0, -1) x (-1, 0, 0)
  circle A0 centre (0, 0) radius 46
  dimension "d208" = 92
  constraints: 1 centre point, 1 coincident
  measures "d208" diameter of A0
extrude "Extrusion30" cut sketch "Sketch34" along normal through all
sketch "Sketch35" plane through (0, 0, 28.9) normal (0, 0, 1) x (1, 0, 0)
  circle A0 centre (0, 0) radius 6.75 projected
  circle A1 centre (0, 0) radius 13 projected
extrude "Extrusion31" add sketch "Sketch35" along normal blind 11.1
sketch "Sketch36" plane through (-52.7965, -12.5, 0) normal (-1, 0, 0) x (0, 0, 1)
  line L0 (34.45, 8.5) -> (40, 8.5) projected
  line L1 (40, 16.5) -> (40, 8.5) projected
  line L2 (40, 16.5) -> (34.45, 16.5) projected
  spline S0 degree 7 poles (34.45, 16.5) (34.0894, 16.5) (33.7292, 16.4621) (33.372, 16.3864) (33.0205, 16.2724) (32.6778, 16.1193) (32.3478, 15.9254) (31.8593, 15.5557) (31.6884, 15.4084) (31.524, 15.247) (31.3675, 15.0712) (31.2201, 14.8807) (31.0836, 14.6751) (30.828, 14.2188) (30.7096, 13.9637) (30.6093, 13.6916) (30.531, 13.4055) (30.4773, 13.1089) (30.45, 12.8058) (30.45, 12.1942) (30.4773, 11.8911) (30.531, 11.5945) (30.6093, 11.3084) (30.7096, 11.0363) (30.828, 10.7812) (31.1347, 10.2336) (31.3351, 9.952) (31.5555, 9.7004) (31.7916, 9.4777) (32.04, 9.2828) (32.2982, 9.1146) (32.8197, 8.8359) (33.0824, 8.7232) (33.3506, 8.6336) (33.6228, 8.5667) (33.8976, 8.5223) (34.1737, 8.5) (34.45, 8.5) knots 0 0 0 0 0 0 0 0 0.230382 0.230382 0.230382 0.230382 0.230382 0.230382 0.360711 0.360711 0.360711 0.360711 0.360711 0.360711 0.49992 0.49992 0.49992 0.49992 0.49992 0.49992 0.639129 0.639129 0.639129 0.639129 0.639129 0.639129 0.823348 0.823348 0.823348 0.823348 0.823348 0.823348 1 1 1 1 1 1 1 1 projected
  point P0 (0, 12.5)
  constraints: 1 vertical alignment
extrude "Extrusion32" add sketch "Sketch36" against normal blind 45
sketch "Sketch37" plane through (0, 0, 10) normal (0, 0, -1) x (-1, 0, 0)
  circle A0 centre (0, 0) radius 11 projected
  circle A1 centre (0, 0) radius 6.75 projected
extrude "Extrusion33" cut sketch "Sketch37" against normal through all
sketch "Sketch38" plane through (0, 0, 25) normal (0, 0, -1) x (-1, 0, 0)
  circle A0 centre (0, 0) radius 11 projected
  circle A1 centre (0, 0) radius 2.5
  dimension "d217" = 5
  constraints: 1 centre point, 1 coincident
  measures "d217" diameter of A1
extrude "Extrusion34" add sketch "Sketch38" against normal blind 15
ref_plane "Work Plane12" through (0, 0, 37) normal (0, 0, 1) x (1, 0, 0)
sketch "Sketch39" plane through (0, 0, 37) normal (0, 0, 1) x (1, 0, 0)
  line L0 (-6.3182, -0.635) -> (-15.3987, -0.635)
  line L1 (-12.5412, 4.8767) -> (-12.5412, 4.7625)
  line L2 (-12.5412, 4.7625) -> (-15.3987, 4.7625)
  line L3 (-15.3987, 4.7625) -> (-15.3987, 0.635)
  line L4 (-15.3987, 0.635) -> (-6.3182, 0.635)
  arc A0 (-6.3182, -0.635) -> (-6.3182, 0.635) centre (0, 0) ccw
  line L5 (-6.3182, -0.635) -> (-15.3987, -0.635)
  line L6 (-15.3987, -0.635) -> (-15.3987, -4.7625)
  line L7 (-15.3987, -4.7625) -> (-13.387, -4.7625)
  arc A1 (-10.2379, -7.4472) -> (-13.387, -4.7625) centre (-13.387, -7.9518) ccw
  arc A2 (-10.2379, -7.4472) -> (-5.4187, -9.9295) centre (-6.9148, -6.9148) ccw
  arc A3 (-2.9466, -9.7233) -> (-5.4187, -9.9295) centre (-3.9227, -12.9442) ccw
  arc A4 (-2.9466, -9.7233) -> (2.9466, -9.7233) centre (0, 0) ccw
  arc A5 (5.4187, -9.9295) -> (2.9466, -9.7233) centre (3.9227, -12.9442) ccw
  arc A6 (5.4187, -9.9295) -> (9.9295, -5.4187) centre (6.9148, -6.9148) ccw
  arc A7 (9.7233, -2.9466) -> (9.9295, -5.4187) centre (12.9442, -3.9227) ccw
  arc A8 (9.7233, -2.9466) -> (9.7233, 2.9466) centre (0, 0) ccw
  arc A9 (9.9295, 5.4187) -> (9.7233, 2.9466) centre (12.9442, 3.9227) ccw
  arc A10 (9.9295, 5.4187) -> (5.4187, 9.9295) centre (6.9148, 6.9148) ccw
  arc A11 (2.9466, 9.7233) -> (5.4187, 9.9295) centre (3.9227, 12.9442) ccw
  arc A12 (2.9466, 9.7233) -> (-2.9466, 9.7233) centre (0, 0) ccw
  arc A13 (-5.4187, 9.9295) -> (-2.9466, 9.7233) centre (-3.9227, 12.9442) ccw
  arc A14 (-5.4187, 9.9295) -> (-10.2379, 7.4472) centre (-6.9148, 6.9148) ccw
  arc A15 (-12.5412, 4.8767) -> (-10.2379, 7.4472) centre (-13.387, 7.9518) ccw
  arc A16 (-5.1647, -7.0079) -> (-5.6245, -5.7287) centre (-6.9148, -6.9148) ccw
  spline S0 degree 3 poles (-5.1647, -7.0079) (-5.1894, -7.1421) (-5.23, -7.2729) (-5.3413, -7.521) (-5.4112, -7.6376) (-5.5805, -7.8561) (-5.7275, -8.0208) (-6.112, -8.2422) (-6.2848, -8.3032) (-6.6088, -8.3538) (-6.7556, -8.3548) (-7.043, -8.3138) (-7.1898, -8.273) (-7.3308, -8.2018) knots 0 0 0 0 0.20469 0.20469 0.40796 0.40796 0.619218 0.619218 0.76586 0.76586 0.883721 0.883721 1 1 1 1
  arc A17 (-8.0559, -6.1887) -> (-7.3308, -8.2018) centre (-6.9148, -6.9148) ccw
  spline S1 degree 3 poles (-8.0559, -6.1887) (-7.9865, -6.0292) (-7.8926, -5.9046) (-7.7117, -5.7056) (-7.5983, -5.6128) (-7.3161, -5.4444) (-7.1433, -5.3807) (-6.7036, -5.3054) (-6.4847, -5.339) (-6.2129, -5.4009) (-6.0851, -5.4464) (-5.8424, -5.5669) (-5.7285, -5.6415) (-5.6245, -5.7287) knots 0 0 0 0 0.10155 0.10155 0.221851 0.221851 0.372602 0.372602 0.589778 0.589778 0.794575 0.794575 1 1 1 1
  arc A18 (5.1647, 7.0079) -> (5.6245, 5.7287) centre (6.9148, 6.9148) ccw
  spline S2 degree 3 poles (5.1647, 7.0079) (5.1894, 7.1421) (5.23, 7.2729) (5.3413, 7.521) (5.4112, 7.6376) (5.5805, 7.8561) (5.7275, 8.0208) (6.112, 8.2422) (6.2848, 8.3032) (6.6088, 8.3538) (6.7556, 8.3548) (7.043, 8.3138) (7.1898, 8.273) (7.3308, 8.2018) knots 0 0 0 0 0.20469 0.20469 0.40796 0.40796 0.619218 0.619218 0.76586 0.76586 0.883721 0.883721 1 1 1 1
  arc A19 (8.0559, 6.1887) -> (7.3308, 8.2018) centre (6.9148, 6.9148) ccw
  spline S3 degree 3 poles (8.0559, 6.1887) (7.9865, 6.0292) (7.8926, 5.9046) (7.7117, 5.7056) (7.5983, 5.6128) (7.3161, 5.4444) (7.1433, 5.3807) (6.7036, 5.3054) (6.4847, 5.339) (6.2129, 5.4009) (6.0851, 5.4464) (5.8424, 5.5669) (5.7285, 5.6415) (5.6245, 5.7287) knots 0 0 0 0 0.10155 0.10155 0.221851 0.221851 0.372602 0.372602 0.589778 0.589778 0.794575 0.794575 1 1 1 1
  arc A20 (-7.0079, 5.1647) -> (-5.7287, 5.6245) centre (-6.9148, 6.9148) ccw
  spline S4 degree 3 poles (-7.0079, 5.1647) (-7.1421, 5.1894) (-7.2729, 5.23) (-7.521, 5.3413) (-7.6376, 5.4112) (-7.8561, 5.5805) (-8.0208, 5.7275) (-8.2422, 6.112) (-8.3032, 6.2848) (-8.3538, 6.6088) (-8.3548, 6.7556) (-8.3138, 7.043) (-8.273, 7.1898) (-8.2018, 7.3308) knots 0 0 0 0 0.20469 0.20469 0.40796 0.40796 0.619218 0.619218 0.76586 0.76586 0.883721 0.883721 1 1 1 1
  arc A21 (-6.1887, 8.0559) -> (-8.2018, 7.3308) centre (-6.9148, 6.9148) ccw
  spline S5 degree 3 poles (-6.1887, 8.0559) (-6.0292, 7.9865) (-5.9046, 7.8926) (-5.7056, 7.7117) (-5.6128, 7.5983) (-5.4444, 7.3161) (-5.3807, 7.1433) (-5.3054, 6.7036) (-5.339, 6.4847) (-5.4009, 6.2129) (-5.4464, 6.0851) (-5.5669, 5.8424) (-5.6415, 5.7285) (-5.7287, 5.6245) knots 0 0 0 0 0.10155 0.10155 0.221851 0.221851 0.372602 0.372602 0.589778 0.589778 0.794575 0.794575 1 1 1 1
  arc A22 (7.0079, -5.1647) -> (5.7287, -5.6245) centre (6.9148, -6.9148) ccw
  spline S6 degree 3 poles (7.0079, -5.1647) (7.1421, -5.1894) (7.2729, -5.23) (7.521, -5.3413) (7.6376, -5.4112) (7.8561, -5.5805) (8.0208, -5.7275) (8.2422, -6.112) (8.3032, -6.2848) (8.3538, -6.6088) (8.3548, -6.7556) (8.3138, -7.043) (8.273, -7.1898) (8.2018, -7.3308) knots 0 0 0 0 0.20469 0.20469 0.40796 0.40796 0.619218 0.619218 0.76586 0.76586 0.883721 0.883721 1 1 1 1
  arc A23 (6.1887, -8.0559) -> (8.2018, -7.3308) centre (6.9148, -6.9148) ccw
  spline S7 degree 3 poles (6.1887, -8.0559) (6.0292, -7.9865) (5.9046, -7.8926) (5.7056, -7.7117) (5.6128, -7.5983) (5.4444, -7.3161) (5.3807, -7.1433) (5.3054, -6.7036) (5.339, -6.4847) (5.4009, -6.2129) (5.4464, -6.0851) (5.5669, -5.8424) (5.6415, -5.7285) (5.7287, -5.6245) knots 0 0 0 0 0.10155 0.10155 0.221851 0.221851 0.372602 0.372602 0.589778 0.589778 0.794575 0.794575 1 1 1 1
  constraints: 48 point on circle, 24 centre point, 16 end point, 16 other
extrude "Extrusion35" cut sketch "Sketch39" against normal blind 15.1
sketch "Sketch40" plane through (0, 0, 25) normal (0, 0, -1) x (-1, 0, 0)
  spline S0 degree 4 poles (6.1887, 8.0559) (6.0952, 8.0152) (6.0065, 7.9643) (5.9231, 7.9048) (5.8372, 7.8309) (5.8287, 7.8234) (5.8204, 7.816) (5.7593, 7.7604) (5.7095, 7.7087) (5.663, 7.654) (5.516, 7.4559) (5.4339, 7.2988) (5.3779, 7.1307) (5.3234, 6.8056) (5.3189, 6.6495) (5.3366, 6.4947) (5.416, 6.1466) (5.4924, 5.9559) (5.5983, 5.7799) (5.7287, 5.6245) knots 0 0 0 0 0 0.135007 0.135007 0.135007 0.150303 0.150303 0.150303 0.250972 0.250972 0.250972 0.496798 0.496798 0.496798 0.714057 0.714057 0.714057 1 1 1 1 1 projected
  arc A0 (5.7287, 5.6245) -> (7.0079, 5.1647) centre (6.9148, 6.9148) ccw projected
  spline S1 degree 4 poles (7.0079, 5.1647) (7.2029, 5.2006) (7.3923, 5.2666) (7.5691, 5.3615) (7.8539, 5.5765) (7.9724, 5.6888) (8.0726, 5.8169) (8.2419, 6.1122) (8.306, 6.2818) (8.3414, 6.4597) (8.3544, 6.8171) (8.3317, 6.9963) (8.2824, 7.1712) (8.2018, 7.3308) knots 0 0 0 0 0 0.279943 0.279943 0.279943 0.503891 0.503891 0.503891 0.752167 0.752167 0.752167 1 1 1 1 1 projected
  arc A1 (8.2018, 7.3308) -> (6.1887, 8.0559) centre (6.9148, 6.9148) ccw projected
  arc A2 (5.6245, -5.7287) -> (5.1647, -7.0079) centre (6.9148, -6.9148) ccw projected
  spline S2 degree 4 poles (5.1647, -7.0079) (5.2006, -7.2029) (5.2666, -7.3923) (5.3615, -7.5691) (5.5765, -7.8539) (5.6888, -7.9724) (5.8169, -8.0726) (6.1122, -8.2419) (6.2818, -8.306) (6.4597, -8.3414) (6.8171, -8.3544) (6.9963, -8.3317) (7.1712, -8.2824) (7.3308, -8.2018) knots 0 0 0 0 0 0.279943 0.279943 0.279943 0.503891 0.503891 0.503891 0.752167 0.752167 0.752167 1 1 1 1 1 projected
  arc A3 (7.3308, -8.2018) -> (8.0559, -6.1887) centre (6.9148, -6.9148) ccw projected
  spline S3 degree 4 poles (8.0559, -6.1887) (8.0152, -6.0952) (7.9643, -6.0065) (7.9048, -5.9231) (7.8309, -5.8372) (7.8234, -5.8287) (7.816, -5.8204) (7.7604, -5.7593) (7.7087, -5.7095) (7.654, -5.663) (7.4559, -5.516) (7.2988, -5.4339) (7.1307, -5.3779) (6.8056, -5.3234) (6.6495, -5.3189) (6.4947, -5.3366) (6.1466, -5.416) (5.9559, -5.4924) (5.7799, -5.5983) (5.6245, -5.7287) knots 0 0 0 0 0 0.135007 0.135007 0.135007 0.150303 0.150303 0.150303 0.250972 0.250972 0.250972 0.496798 0.496798 0.496798 0.714057 0.714057 0.714057 1 1 1 1 1 projected
  spline S4 degree 4 poles (-6.1887, -8.0559) (-6.0952, -8.0152) (-6.0065, -7.9643) (-5.9231, -7.9048) (-5.8372, -7.8309) (-5.8287, -7.8234) (-5.8204, -7.816) (-5.7593, -7.7604) (-5.7095, -7.7087) (-5.663, -7.654) (-5.516, -7.4559) (-5.4339, -7.2988) (-5.3779, -7.1307) (-5.3234, -6.8056) (-5.3189, -6.6495) (-5.3366, -6.4947) (-5.416, -6.1466) (-5.4924, -5.9559) (-5.5983, -5.7799) (-5.7287, -5.6245) knots 0 0 0 0 0 0.135007 0.135007 0.135007 0.150303 0.150303 0.150303 0.250972 0.250972 0.250972 0.496798 0.496798 0.496798 0.714057 0.714057 0.714057 1 1 1 1 1 projected
  arc A4 (-5.7287, -5.6245) -> (-7.0079, -5.1647) centre (-6.9148, -6.9148) ccw projected
  spline S5 degree 4 poles (-7.0079, -5.1647) (-7.2029, -5.2006) (-7.3923, -5.2666) (-7.5691, -5.3615) (-7.8539, -5.5765) (-7.9724, -5.6888) (-8.0726, -5.8169) (-8.2419, -6.1122) (-8.306, -6.2818) (-8.3414, -6.4597) (-8.3544, -6.8171) (-8.3317, -6.9963) (-8.2824, -7.1712) (-8.2018, -7.3308) knots 0 0 0 0 0 0.279943 0.279943 0.279943 0.503891 0.503891 0.503891 0.752167 0.752167 0.752167 1 1 1 1 1 projected
  arc A5 (-8.2018, -7.3308) -> (-6.1887, -8.0559) centre (-6.9148, -6.9148) ccw projected
  spline S6 degree 4 poles (-5.1647, 7.0079) (-5.2006, 7.2029) (-5.2666, 7.3923) (-5.3615, 7.5691) (-5.5765, 7.8539) (-5.6888, 7.9724) (-5.8169, 8.0726) (-6.1122, 8.2419) (-6.2818, 8.306) (-6.4597, 8.3414) (-6.8171, 8.3544) (-6.9963, 8.3317) (-7.1712, 8.2824) (-7.3308, 8.2018) knots 0 0 0 0 0 0.279943 0.279943 0.279943 0.503891 0.503891 0.503891 0.752167 0.752167 0.752167 1 1 1 1 1 projected
  arc A6 (-7.3308, 8.2018) -> (-8.0559, 6.1887) centre (-6.9148, 6.9148) ccw projected
  spline S7 degree 4 poles (-8.0559, 6.1887) (-8.0152, 6.0952) (-7.9643, 6.0065) (-7.9048, 5.9231) (-7.8309, 5.8372) (-7.8234, 5.8287) (-7.816, 5.8204) (-7.7604, 5.7593) (-7.7087, 5.7095) (-7.654, 5.663) (-7.4559, 5.516) (-7.2988, 5.4339) (-7.1307, 5.3779) (-6.8056, 5.3234) (-6.6495, 5.3189) (-6.4947, 5.3366) (-6.1466, 5.416) (-5.9559, 5.4924) (-5.7799, 5.5983) (-5.6245, 5.7287) knots 0 0 0 0 0 0.135007 0.135007 0.135007 0.150303 0.150303 0.150303 0.250972 0.250972 0.250972 0.496798 0.496798 0.496798 0.714057 0.714057 0.714057 1 1 1 1 1 projected
  arc A7 (-5.6245, 5.7287) -> (-5.1647, 7.0079) centre (-6.9148, 6.9148) ccw projected
  circle A8 centre (0, 0) radius 2.5 projected
  circle A9 centre (0, 0) radius 6.35
  dimension "d223" = 12.7
  constraints: 1 centre point, 1 coincident, 8 other
  measures "d223" diameter of A9
extrude "Extrusion36" cut sketch "Sketch40" against normal through all contours A1 S1 A0 S0 | S3 A3 S2 A2 | A5 S5 A4 S4 | A7 S7 A6 S6 | A8 | A9
sketch "Sketch41" plane through (0, 0, 37) normal (0, 0, -1) x (-1, 0, 0)
  spline S0 degree 3 poles (6.1887, 8.0559) (6.0292, 7.9865) (5.9046, 7.8926) (5.7056, 7.7117) (5.6128, 7.5983) (5.4444, 7.3161) (5.3807, 7.1433) (5.3054, 6.7036) (5.339, 6.4847) (5.4009, 6.2129) (5.4464, 6.0851) (5.5669, 5.8424) (5.6415, 5.7285) (5.7287, 5.6245) knots 0 0 0 0 0.10155 0.10155 0.221851 0.221851 0.372602 0.372602 0.589778 0.589778 0.794575 0.794575 1 1 1 1 projected
  arc A0 (8.2018, 7.3308) -> (6.1887, 8.0559) centre (6.9148, 6.9148) ccw projected
  spline S1 degree 3 poles (7.0079, 5.1647) (7.1421, 5.1894) (7.2729, 5.23) (7.521, 5.3413) (7.6376, 5.4112) (7.8561, 5.5805) (8.0208, 5.7275) (8.2422, 6.112) (8.3032, 6.2848) (8.3538, 6.6088) (8.3548, 6.7556) (8.3138, 7.043) (8.273, 7.1898) (8.2018, 7.3308) knots 0 0 0 0 0.20469 0.20469 0.40796 0.40796 0.619218 0.619218 0.76586 0.76586 0.883721 0.883721 1 1 1 1 projected
  arc A1 (5.7287, 5.6245) -> (7.0079, 5.1647) centre (6.9148, 6.9148) ccw projected
  spline S2 degree 3 poles (-6.1887, -8.0559) (-6.0292, -7.9865) (-5.9046, -7.8926) (-5.7056, -7.7117) (-5.6128, -7.5983) (-5.4444, -7.3161) (-5.3807, -7.1433) (-5.3054, -6.7036) (-5.339, -6.4847) (-5.4009, -6.2129) (-5.4464, -6.0851) (-5.5669, -5.8424) (-5.6415, -5.7285) (-5.7287, -5.6245) knots 0 0 0 0 0.10155 0.10155 0.221851 0.221851 0.372602 0.372602 0.589778 0.589778 0.794575 0.794575 1 1 1 1 projected
  arc A2 (-8.2018, -7.3308) -> (-6.1887, -8.0559) centre (-6.9148, -6.9148) ccw projected
  spline S3 degree 3 poles (-7.0079, -5.1647) (-7.1421, -5.1894) (-7.2729, -5.23) (-7.521, -5.3413) (-7.6376, -5.4112) (-7.8561, -5.5805) (-8.0208, -5.7275) (-8.2422, -6.112) (-8.3032, -6.2848) (-8.3538, -6.6088) (-8.3548, -6.7556) (-8.3138, -7.043) (-8.273, -7.1898) (-8.2018, -7.3308) knots 0 0 0 0 0.20469 0.20469 0.40796 0.40796 0.619218 0.619218 0.76586 0.76586 0.883721 0.883721 1 1 1 1 projected
  arc A3 (-5.7287, -5.6245) -> (-7.0079, -5.1647) centre (-6.9148, -6.9148) ccw projected
  spline S4 degree 3 poles (-5.1647, 7.0079) (-5.1894, 7.1421) (-5.23, 7.2729) (-5.3413, 7.521) (-5.4112, 7.6376) (-5.5805, 7.8561) (-5.7275, 8.0208) (-6.112, 8.2422) (-6.2848, 8.3032) (-6.6088, 8.3538) (-6.7556, 8.3548) (-7.043, 8.3138) (-7.1898, 8.273) (-7.3308, 8.2018) knots 0 0 0 0 0.20469 0.20469 0.40796 0.40796 0.619218 0.619218 0.76586 0.76586 0.883721 0.883721 1 1 1 1 projected
  arc A4 (-5.6245, 5.7287) -> (-5.1647, 7.0079) centre (-6.9148, 6.9148) ccw projected
  spline S5 degree 3 poles (-8.0559, 6.1887) (-7.9865, 6.0292) (-7.8926, 5.9046) (-7.7117, 5.7056) (-7.5983, 5.6128) (-7.3161, 5.4444) (-7.1433, 5.3807) (-6.7036, 5.3054) (-6.4847, 5.339) (-6.2129, 5.4009) (-6.0851, 5.4464) (-5.8424, 5.5669) (-5.7285, 5.6415) (-5.6245, 5.7287) knots 0 0 0 0 0.10155 0.10155 0.221851 0.221851 0.372602 0.372602 0.589778 0.589778 0.794575 0.794575 1 1 1 1 projected
  arc A5 (-7.3308, 8.2018) -> (-8.0559, 6.1887) centre (-6.9148, 6.9148) ccw projected
  arc A6 (5.6245, -5.7287) -> (5.1647, -7.0079) centre (6.9148, -6.9148) ccw projected
  spline S6 degree 3 poles (8.0559, -6.1887) (7.9865, -6.0292) (7.8926, -5.9046) (7.7117, -5.7056) (7.5983, -5.6128) (7.3161, -5.4444) (7.1433, -5.3807) (6.7036, -5.3054) (6.4847, -5.339) (6.2129, -5.4009) (6.0851, -5.4464) (5.8424, -5.5669) (5.7285, -5.6415) (5.6245, -5.7287) knots 0 0 0 0 0.10155 0.10155 0.221851 0.221851 0.372602 0.372602 0.589778 0.589778 0.794575 0.794575 1 1 1 1 projected
  arc A7 (7.3308, -8.2018) -> (8.0559, -6.1887) centre (6.9148, -6.9148) ccw projected
  spline S7 degree 3 poles (5.1647, -7.0079) (5.1894, -7.1421) (5.23, -7.2729) (5.3413, -7.521) (5.4112, -7.6376) (5.5805, -7.8561) (5.7275, -8.0208) (6.112, -8.2422) (6.2848, -8.3032) (6.6088, -8.3538) (6.7556, -8.3548) (7.043, -8.3138) (7.1898, -8.273) (7.3308, -8.2018) knots 0 0 0 0 0.20469 0.20469 0.40796 0.40796 0.619218 0.619218 0.76586 0.76586 0.883721 0.883721 1 1 1 1 projected
  arc A8 (5.4187, -9.9295) -> (10.2379, -7.4472) centre (6.9148, -6.9148) ccw projected
  arc A9 (13.387, -4.7625) -> (10.2379, -7.4472) centre (13.387, -7.9518) ccw projected
  line L0 (13.387, -4.7625) -> (15.3987, -4.7625) projected
  line L1 (15.3987, -4.7625) -> (15.3987, -0.635) projected
  line L2 (15.3987, -0.635) -> (6.3182, -0.635) projected
  arc A10 (6.3182, 0.635) -> (6.3182, -0.635) centre (0, 0) ccw projected
  line L3 (6.3182, 0.635) -> (15.3987, 0.635) projected
  line L4 (15.3987, 0.635) -> (15.3987, 4.7625) projected
  line L5 (15.3987, 4.7625) -> (12.5412, 4.7625) projected
  line L6 (12.5412, 4.7625) -> (12.5412, 4.8767) projected
  arc A11 (10.2379, 7.4472) -> (12.5412, 4.8767) centre (13.387, 7.9518) ccw projected
  arc A12 (10.2379, 7.4472) -> (5.4187, 9.9295) centre (6.9148, 6.9148) ccw projected
  arc A13 (2.9466, 9.7233) -> (5.4187, 9.9295) centre (3.9227, 12.9442) ccw projected
  arc A14 (2.9466, 9.7233) -> (-2.9466, 9.7233) centre (0, 0) ccw projected
  arc A15 (-5.4187, 9.9295) -> (-2.9466, 9.7233) centre (-3.9227, 12.9442) ccw projected
  arc A16 (-5.4187, 9.9295) -> (-9.9295, 5.4187) centre (-6.9148, 6.9148) ccw projected
  arc A17 (-9.7233, 2.9466) -> (-9.9295, 5.4187) centre (-12.9442, 3.9227) ccw projected
  arc A18 (-9.7233, 2.9466) -> (-9.7233, -2.9466) centre (0, 0) ccw projected
  arc A19 (-9.9295, -5.4187) -> (-9.7233, -2.9466) centre (-12.9442, -3.9227) ccw projected
  arc A20 (-9.9295, -5.4187) -> (-5.4187, -9.9295) centre (-6.9148, -6.9148) ccw projected
  arc A21 (-2.9466, -9.7233) -> (-5.4187, -9.9295) centre (-3.9227, -12.9442) ccw projected
  arc A22 (-2.9466, -9.7233) -> (2.9466, -9.7233) centre (0, 0) ccw projected
  arc A23 (5.4187, -9.9295) -> (2.9466, -9.7233) centre (3.9227, -12.9442) ccw projected
  line L7 (6.9148, 6.9148) -> (6.9148, 10.2803)
  arc A24 (10.2379, 7.4472) -> (5.4187, 9.9295) centre (6.9148, 6.9148) ccw projected
  line L8 (6.9148, 10.2803) -> (15.3987, 10.2803)
  line L9 (15.3987, 10.2803) -> (15.3987, -10.2803)
  line L10 (15.3987, -10.2803) -> (6.9148, -10.2803)
  arc A25 (5.4187, -9.9295) -> (10.2379, -7.4472) centre (6.9148, -6.9148) ccw projected
  line L11 (6.9148, -6.9148) -> (6.9148, -10.2803)
  line L12 (6.9148, -6.9148) -> (6.9148, 6.9148)
  point P0 (15.3987, 2.6988)
  constraints: 12 end point, 4 point on circle, 3 vertical, 2 horizontal, 1 midpoint, 1 parallel, 1 point on line, 8 other
extrude "Extrusion37" cut sketch "Sketch41" along normal through all contours S0 A1 L12 L3 A10 L2 S6 A6 S7 L11 A8 A23 A22 A21 A20 A19 A18 A17 A16 A15 A14 A13 A12 L7 A0 | L7 A12 A11 L6 L5 L4 L3 L12 A1 S1 A0 | L8 L9 L5 L6 A11 A12 | L12 L2 A10 L3 | L3 L9 L2 L12 | L2 L1 L0 A9 A8 L11 S7 A7 S6 L12 | L9 L10 A8 A9 L0
sketch "Sketch42" plane through (0, 0, 37) normal (0, 0, -1) x (-1, 0, 0)
  circle A0 centre (0, 0) radius 6.35 projected
  arc A1 (8.2018, 7.3308) -> (6.1887, 8.0559) centre (6.9148, 6.9148) ccw projected
  arc A2 (5.7287, 5.6245) -> (7.0079, 5.1647) centre (6.9148, 6.9148) ccw projected
  arc A3 (-8.2018, -7.3308) -> (-6.1887, -8.0559) centre (-6.9148, -6.9148) ccw projected
  arc A4 (-5.7287, -5.6245) -> (-7.0079, -5.1647) centre (-6.9148, -6.9148) ccw projected
  arc A5 (-5.6245, 5.7287) -> (-5.1647, 7.0079) centre (-6.9148, 6.9148) ccw projected
  arc A6 (-7.3308, 8.2018) -> (-8.0559, 6.1887) centre (-6.9148, 6.9148) ccw projected
  arc A7 (5.6245, -5.7287) -> (5.1647, -7.0079) centre (6.9148, -6.9148) ccw projected
  arc A8 (7.3308, -8.2018) -> (8.0559, -6.1887) centre (6.9148, -6.9148) ccw projected
  line L0 (15.3987, -10.2803) -> (15.3987, 10.2803) projected
  line L1 (15.3987, 10.2803) -> (6.9148, 10.2803) projected
  arc A9 (6.9148, 10.2803) -> (5.4187, 9.9295) centre (6.9148, 6.9148) ccw projected
  arc A10 (2.9466, 9.7233) -> (5.4187, 9.9295) centre (3.9227, 12.9442) ccw projected
  arc A11 (2.9466, 9.7233) -> (-2.9466, 9.7233) centre (0, 0) ccw projected
  arc A12 (-5.4187, 9.9295) -> (-2.9466, 9.7233) centre (-3.9227, 12.9442) ccw projected
  arc A13 (-5.4187, 9.9295) -> (-9.9295, 5.4187) centre (-6.9148, 6.9148) ccw projected
  arc A14 (-9.7233, 2.9466) -> (-9.9295, 5.4187) centre (-12.9442, 3.9227) ccw projected
  arc A15 (-9.7233, 2.9466) -> (-9.7233, -2.9466) centre (0, 0) ccw projected
  arc A16 (-9.9295, -5.4187) -> (-9.7233, -2.9466) centre (-12.9442, -3.9227) ccw projected
  arc A17 (-9.9295, -5.4187) -> (-5.4187, -9.9295) centre (-6.9148, -6.9148) ccw projected
  arc A18 (-2.9466, -9.7233) -> (-5.4187, -9.9295) centre (-3.9227, -12.9442) ccw projected
  arc A19 (-2.9466, -9.7233) -> (2.9466, -9.7233) centre (0, 0) ccw projected
  arc A20 (5.4187, -9.9295) -> (2.9466, -9.7233) centre (3.9227, -12.9442) ccw projected
  arc A21 (5.4187, -9.9295) -> (6.9148, -10.2803) centre (6.9148, -6.9148) ccw projected
  line L2 (6.9148, -10.2803) -> (15.3987, -10.2803) projected
  line L3 (17.3987, 12.2803) -> (17.3987, -12.2803)
  line L4 (17.3987, -12.2803) -> (6.9148, -12.2803)
  arc A22 (4.5297, -11.721) -> (6.9148, -12.2803) centre (6.9148, -6.9148) ccw
  arc A23 (4.5297, -11.721) -> (3.5266, -11.6374) centre (3.9227, -12.9442) ccw
  arc A24 (-3.5266, -11.6374) -> (3.5266, -11.6374) centre (0, 0) ccw
  arc A25 (-3.5266, -11.6374) -> (-4.5297, -11.721) centre (-3.9227, -12.9442) ccw
  arc A26 (-11.721, -4.5297) -> (-4.5297, -11.721) centre (-6.9148, -6.9148) ccw
  arc A27 (-11.721, -4.5297) -> (-11.6374, -3.5266) centre (-12.9442, -3.9227) ccw
  arc A28 (-11.6374, 3.5266) -> (-11.6374, -3.5266) centre (0, 0) ccw
  arc A29 (-11.6374, 3.5266) -> (-11.721, 4.5297) centre (-12.9442, 3.9227) ccw
  arc A30 (-4.5297, 11.721) -> (-11.721, 4.5297) centre (-6.9148, 6.9148) ccw
  arc A31 (-4.5297, 11.721) -> (-3.5266, 11.6374) centre (-3.9227, 12.9442) ccw
  arc A32 (3.5266, 11.6374) -> (-3.5266, 11.6374) centre (0, 0) ccw
  arc A33 (3.5266, 11.6374) -> (4.5297, 11.721) centre (3.9227, 12.9442) ccw
  arc A34 (6.9148, 12.2803) -> (4.5297, 11.721) centre (6.9148, 6.9148) ccw
  line L5 (6.9148, 12.2803) -> (17.3987, 12.2803)
  dimension "d228" = 2
  constraints: 26 point on circle, 13 centre point, 6 end point, 23 other
  measures "d228" distance between parallel lines of L0 L3
extrude "Extrusion38" cut sketch "Sketch42" along normal through all contours A0 | L2 A21 A20 A19 A18 A17 A16 A15 A14 A13 A12 A11 A10 A9 L1 L0 | L3 L4 A22 A23 A24 A25 A26 A27 A28 A29 A30 A31 A32 A33 A34 L5
equation "\"d0\" = 1.1 * da_df"
equation "\"d1\" = da_b"
equation "\"d3\" = da_dw"
equation "\"da_df\" = 95"
equation "\"da_b\" = 10"
equation "\"da_dw\" = 90"
body "Solid1"
body "Srf1"
